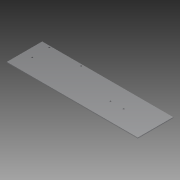
# Autodesk Inventor part: Mounting Board 2
Saved by Autodesk Inventor 2013 (Build 170138000, 138)
## iProperties
Created: 2013-01-26
Part Number: Mounting Board 2
Material: Polycarbonate, Clear
Document SubType Name: Modeling
Designer: Moses
Mass: 202.404 g
Surface Area: 1099.7 cm^2
Volume: 168.67 cm^3
Density: 1.2 g/cm^3
Author: Moses
Autodesk Inventor part; units mm, degrees
ref_plane "YZ Plane" through (0, 0, 0) normal (1, 0, 0) x (0, 1, 0)
ref_plane "XZ Plane" through (0, 0, 0) normal (0, 1, 0) x (-1, 0, 0)
ref_plane "XY Plane" through (0, 0, 0) normal (0, 0, 1) x (1, 0, 0)
sketch "Sketch1" plane through (0, 0, 0) normal (0, 1, 0) x (-1, 0, 0)
  line L0 (0, 0) -> (469.9, 0)
  line L1 (469.9, 0) -> (469.9, 127)
  line L2 (469.9, 127) -> (0, 127)
  line L3 (0, 127) -> (0, 0)
  circle A0 centre (323.85, 6.35) radius 2.54
  line L4 (323.85, 6.35) -> (438.15, 6.35) construction
  circle A1 centre (438.15, 6.35) radius 2.54
  line L5 (438.15, 6.35) -> (438.15, 67.31) construction
  circle A2 centre (438.15, 67.31) radius 2.54
  line L6 (114.3, 63.5) -> (161.544, 63.5) construction
  circle A3 centre (114.3, 63.5) radius 2.54
  circle A4 centre (161.544, 63.5) radius 2.54
  dimension "d0" = 469.9
  dimension "d2" = 127
  dimension "d3" = 5.08
  dimension "d4" = 114.3
  dimension "d5" = 60.96
  dimension "d6" = 31.75
  dimension "d7" = 6.35
  dimension "d8" = 47.244
  dimension "d9" = 5.08
  dimension "d10" = 63.5
  dimension "d11" = 114.3
  constraints: 14 end point, 5 centre point, 4 coincident, 4 perpendicular, 3 equal radius, 2 parallel, 1 horizontal
  measures "d0" distance of L1.end L2.end
  measures "d2" distance of L0.end L1.end
  measures "d3" diameter of A0
  measures "d4" distance of L4.start L4.end
  measures "d5" distance of L5.start L5.end
  measures "d6" distance between parallel lines of L1 L5
  measures "d7" distance between parallel lines of L0 L4
  measures "d8" distance of L6.start L6.end
  measures "d9" diameter of A3
  measures "d10" distance between parallel lines of L0 L6
  measures "d11" distance from line of L6.start L3
extrude "Extrusion1" add sketch "Sketch1" along normal blind 3.175
body "Solid1"
